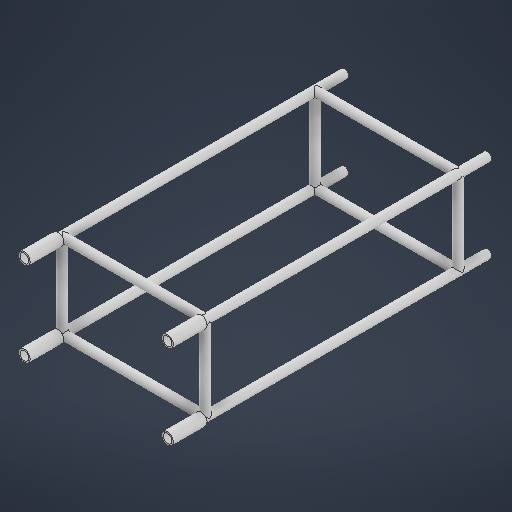
# Autodesk Inventor part: RCPlaneSkeletonMiddleBack2
Saved by Autodesk Inventor 2026.1 (Build 301233000, 233)
## iProperties
Created: 2026-03-03
Part Number: RCPlaneSkeletonMiddleBack2
Material: Generic
Document SubType Name: Modeling
Designer: morri
Density: 1 g/cm^3
Appearance: Default
Author: morri
Autodesk Inventor part; units mm, degrees
ref_plane "YZ Plane" through (0, 0, 0) normal (1, 0, 0) x (0, 1, 0)
ref_plane "XZ Plane" through (0, 0, 0) normal (0, 1, 0) x (-1, 0, 0)
ref_plane "XY Plane" through (0, 0, 0) normal (0, 0, 1) x (1, 0, 0)
sketch "Sketch1" plane through (0, 0, 0) normal (0, 0, 1) x (1, 0, 0)
  line L0 (0, 0) -> (85, 0) construction
  line L1 (85, 0) -> (85, 50) construction
  line L2 (85, 50) -> (0, 50) construction
  line L3 (0, 50) -> (0, 0) construction
  circle A0 centre (0, 0) radius 2.5
  circle A1 centre (0, 50) radius 2.5
  circle A2 centre (85, 50) radius 2.5
  circle A3 centre (85, 0) radius 2.5
  dimension "d0" = 85
  dimension "d1" = 50
  dimension "d2" = 5
  dimension "d3" = 5
  dimension "d4" = 5
  dimension "d5" = 5
  constraints: 8 end point, 4 centre point, 4 coincident, 2 parallel, 1 horizontal, 1 perpendicular
  measures "d0" distance of L2.end L1.end
  measures "d1" distance of L1.end L0.end
  measures "d2" diameter of A0
  measures "d3" diameter of A1
  measures "d4" diameter of A2
  measures "d5" diameter of A3
extrude "Length Beams" add sketch "Sketch1" along normal blind 150
sketch "Sketch2" plane through (0, 0, 0) normal (0, 1, 0) x (-1, 0, 0)
  circle A0 centre (0, 0) radius 2.5
  line L0 (-82.5, 0) -> (-87.5, 0) projected
  circle A1 centre (-85, 0) radius 2.5
  line L1 (2.5, 150) -> (-2.5, 150) projected
  circle A2 centre (0, 150) radius 2.5
  line L2 (-82.5, 150) -> (-87.5, 150) projected
  circle A3 centre (-85, 150) radius 2.5
  dimension "d8" = 5
  dimension "d9" = 5
  dimension "d10" = 5
  dimension "d11" = 5
  constraints: 4 centre point, 3 midpoint, 1 coincident
  measures "d8" diameter of A0
  measures "d9" diameter of A1
  measures "d10" diameter of A2
  measures "d11" diameter of A3
extrude "Vertical Beam" add sketch "Sketch2" along normal blind 50
sketch "Sketch3" plane through (0, 0, 0) normal (1, 0, 0) x (0, 1, 0)
  circle A0 centre (50, 0) radius 2.5
  circle A1 centre (0, 0) radius 2.5
  circle A2 centre (0, 150) radius 2.5
  line L0 (50, 150) -> (50, 152.5) projected
  circle A3 centre (50, 150) radius 2.5
  dimension "d14" = 5
  dimension "d15" = 5
  dimension "d16" = 5
  dimension "d17" = 5
  constraints: 4 centre point, 1 coincident
  measures "d14" diameter of A0
  measures "d15" diameter of A1
  measures "d16" diameter of A2
  measures "d17" diameter of A3
extrude "Width Beams" add sketch "Sketch3" along normal blind 85
sketch "Sketch4" plane through (0, 0, 150) normal (0, 0, 1) x (1, 0, 0)
  arc A0 (0, 52.5) -> (-2.5, 50) centre (0, 50) ccw projected
  circle A1 centre (0, 50) radius 2.5
  line L0 (82.5, 47.5) -> (85, 50) projected
  circle A2 centre (85, 50) radius 2.5
  arc A3 (87.5, 0) -> (83.2322, 1.7678) centre (85, 0) ccw projected
  circle A4 centre (85, 0) radius 2.5
  circle A5 centre (0, 0) radius 2.5
  point P0 (83.2322, 48.2322)
  point P1 (83.2322, 1.7678)
  dimension "d20" = 5
  dimension "d21" = 5
  dimension "d22" = 5
  dimension "d23" = 5
  constraints: 4 centre point, 3 coincident
  measures "d20" diameter of A1
  measures "d21" diameter of A2
  measures "d22" diameter of A4
  measures "d23" diameter of A5
extrude "Female Flush" add sketch "Sketch4" along normal blind 2.5
sketch "Sketch7" plane through (0, 0, 0) normal (0, 0, -1) x (-1, 0, 0)
  circle A0 centre (0, 0) radius 2.5
  arc A1 (-2.5, 50) -> (0, 47.5) centre (0, 50) ccw projected
  circle A2 centre (0, 50) radius 2.5
  arc A3 (-85, 47.5) -> (-82.5, 50) centre (-85, 50) ccw projected
  circle A4 centre (-85, 50) radius 2.5
  circle A5 centre (-85, 0) radius 2.5
  dimension "d40" = 5
  dimension "d41" = 5
  dimension "d42" = 5
  constraints: 4 centre point, 2 coincident
  measures "d40" diameter of A2
  measures "d41" diameter of A4
  measures "d42" diameter of A5
extrude "Male Flush" add sketch "Sketch7" along normal blind 2.5
sketch "Sketch9" plane through (0, 0, -2.5) normal (0, 0, -1) x (-1, 0, 0)
  circle A0 centre (0, 0) radius 2.5
  arc A1 (-1.7678, 48.2322) -> (2.5, 50) centre (0, 50) ccw projected
  circle A2 centre (0, 50) radius 2.5
  arc A3 (-83.2322, 48.2322) -> (-85, 52.5) centre (-85, 50) ccw projected
  circle A4 centre (-85, 50) radius 2.5
  arc A5 (-85, -2.5) -> (-82.5, 0) centre (-85, 0) ccw projected
  circle A6 centre (-85, 0) radius 2.5
  point P0 (2.5, 50)
  point P1 (-1.7678, 48.2322)
  point P2 (-85, 52.5)
  point P3 (-82.5, 0)
  point P4 (-85, -2.5)
  dimension "d45" = 5
  dimension "d46" = 5
  dimension "d47" = 5
  dimension "d48" = 5
  constraints: 4 centre point, 4 coincident
  measures "d45" diameter of A0
  measures "d46" diameter of A2
  measures "d47" diameter of A4
  measures "d48" diameter of A6
extrude "Male Connect" add sketch "Sketch9" along normal blind 15
sketch "Sketch10" plane through (0, 0, 152.5) normal (0, 0, 1) x (1, 0, 0)
  arc A0 (0, 47.5) -> (1.7678, 48.2322) centre (0, 50) ccw projected
  circle A1 centre (0, 50) radius 3.5
  arc A2 (83.2322, 48.2322) -> (87.5, 50) centre (85, 50) ccw projected
  circle A3 centre (85, 50) radius 3.5
  circle A4 centre (0, 0) radius 3.5
  arc A5 (87.5, 0) -> (83.2322, 1.7678) centre (85, 0) ccw projected
  circle A6 centre (85, 0) radius 3.5
  dimension "d51" = 7
  dimension "d52" = 7
  dimension "d62" = 7
  dimension "d63" = 7
  constraints: 4 centre point, 4 coincident
  measures "d51" diameter of A1
  measures "d52" diameter of A3
  measures "d62" diameter of A4
  measures "d63" diameter of A6
extrude "Female Connect Top" add sketch "Sketch10" along normal blind 20 contours A1 | A3
extrude "Extrusion9" add sketch "Sketch10" along normal blind 20 contours A4 | A6
sketch "Sketch12" plane through (0, 0, 172.5) normal (0, 0, 1) x (1, 0, 0)
  arc A0 (0, 47.5) -> (1.7678, 48.2322) centre (0, 50) ccw projected
  arc A1 (81.5, 50) -> (85, 46.5) centre (85, 50) ccw projected
  arc A2 (81.5, 0) -> (85, 3.5) centre (85, 0) ccw projected
  point P0 (0, 0)
  point P1 (0, 0)
  constraints: 4 coincident
hole "Hole3" at (0, 50, 172.5) at (85, 50, 172.5) at (85, 0, 172.5) at (0, 0, 172.5) direction (0, 0, -1) diameter 5.3 depth 15
equation "\"fitTol\" = 0.3"
body "Solid1"
